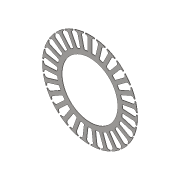
# Autodesk Inventor part: stator-sheet
Saved by Autodesk Inventor 2022 (Build 260153000, 153)
## iProperties
Created: 2025-01-12
Part Number: stator-sheet
Material: Generic
Document SubType Name: Modeling
Designer: Home
Density: 1 g/cm^3
Appearance: Steel - Polished
Author: Home
Autodesk Inventor part; units mm, degrees
ref_plane "YZ Plane" through (0, 0, 0) normal (1, 0, 0) x (0, 1, 0)
ref_plane "XZ Plane" through (0, 0, 0) normal (0, 1, 0) x (-1, 0, 0)
ref_plane "XY Plane" through (0, 0, 0) normal (0, 0, 1) x (1, 0, 0)
sketch "Sketch1" plane through (0, 0, 0) normal (0, 0, 1) x (1, 0, 0)
  circle A0 centre (0, 0) radius 36
  circle A1 centre (0, 0) radius 31
  dimension "d0" = 72
  dimension "d1" = 62
  constraints: 2 centre point, 2 coincident
  measures "d0" diameter of A0
  measures "d1" diameter of A1
extrude "Extrusion1" add sketch "Sketch1" along normal blind 0.5
sketch "Sketch2" plane through (0, 0, 0.5) normal (0, 0, 1) x (1, 0, 0)
  line L0 (0, 0) -> (0, 63.5083) construction
  line L1 (-2, 35.9444) -> (2, 35.9444)
  line L2 (2, 35.9444) -> (2, 52.4619)
  line L3 (2, 52.4619) -> (-2, 52.4619)
  line L4 (-2, 52.4619) -> (-2, 35.9444)
  circle A0 centre (0, 0) radius 36 projected
  circle A1 centre (0, 0) radius 52.5
  circle A2 centre (0, 0) radius 51.5
  circle A3 centre (3, 36.8782) radius 1
  circle A4 centre (-3, 36.8782) radius 1
  circle A5 centre (-4.6341, 48.6457) radius 2.6341
  circle A6 centre (4.6341, 48.6457) radius 2.6341
  line L5 (5, 52.2614) -> (4.8839, 51.2679)
  line L6 (-4.8839, 51.2679) -> (-5, 52.2614)
  point P0 (-2, 36.8782)
  point P1 (-2.9189, 35.8815)
  point P2 (2.9189, 35.8815)
  point P3 (2, 36.8782)
  point P4 (2, 48.6457)
  point P5 (4.7296, 51.2824)
  point P6 (-4.7296, 51.2824)
  point P7 (-2, 48.6457)
  point P8 (2, 52.4619)
  dimension "d5" = 4
  dimension "d6" = 2
  dimension "d7" = 105
  dimension "d8" = 103
  dimension "d9" = 2
  dimension "d10" = 2
  dimension "d13" = 6.667
  dimension "d14" = 6.667
  dimension "d15" = 5
  dimension "d16" = 5
  constraints: 14 end point, 7 point on circle, 4 centre point, 4 tangent, 3 coincident, 3 vertical, 2 parallel, 1 horizontal, 1 perpendicular, 8 other
  measures "d5" distance of L3.end L2.end
  measures "d6" distance between parallel lines of L4 L0
  measures "d7" diameter of A1
  measures "d8" diameter of A2
  measures "d9" diameter of A3
  measures "d10" diameter of A4
  measures "d13" angle of L2 L5
  measures "d14" angle of L4 L6
  measures "d15" distance from line of L0 L6.end
  measures "d16" distance from line of L5.start L0
extrude "Extrusion2" add sketch "Sketch2" against normal blind 0.5 contours A0 L1 | A0 A4 L4 | L4 A2 L2 A0 | L2 A3 A0 | A5 A2 L4 | L2 A2 A6 | A2 L6 A1 L4 | L4 L3 L2 A2 | L2 A1 L5 A2 | A1 L3 picked at (-0.2223, 35.9609)
pattern_circular "Circular Pattern1" count 27 over 360 about axis through (0, 0, 0) along (0, 0, 1) of "Extrusion2"
chamfer "Chamfer1" distance 0.05 angle 45 27 edges at (-23.562, 46.9157, 0.5) (-12.1073, 51.0849, 0.5) (0, 52.5, 0.5) (12.1073, 51.0849, 0.5) (23.562, 46.9157, 0.5) (33.7463, 40.2173, 0.5) (42.1115, 31.3508, 0.5) (48.2063, 20.7942, 0.5) (51.7024, 9.1165, 0.5) (52.4112, -3.0526, 0.5) (50.2944, -15.0572, 0.5) (45.4663, -26.25, 0.5) (38.1871, -36.0277, 0.5) (28.8492, -43.8631, 0.5) (17.9561, -49.3339, 0.5) (6.0949, -52.145, 0.5) (-6.0949, -52.145, 0.5) (-17.9561, -49.3339, 0.5) (-28.8492, -43.8631, 0.5) (-38.1871, -36.0277, 0.5) (-45.4663, -26.25, 0.5) (-50.2944, -15.0572, 0.5) (-52.4112, -3.0526, 0.5) (-51.7024, 9.1165, 0.5) (-48.2063, 20.7942, 0.5) (-42.1115, 31.3508, 0.5) (-33.7463, 40.2173, 0.5)
equation "\"d10\" = d9"
equation "\"d14\" = d13"
equation "\"d16\" = d15"
body "Solid1"
